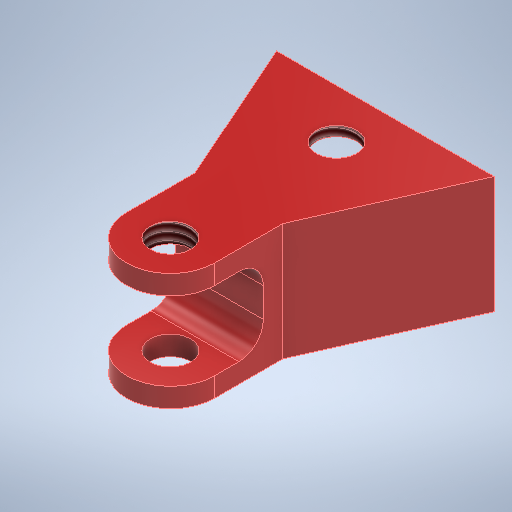
# Autodesk Inventor part: Fixation_rotule_axe_centrale
Saved by Autodesk Inventor 2026.2 (Build 302298010, 298A)
## iProperties
Created: 2026-03-16
Part Number: Fixation_rotule_axe_centrale
Material: Générique
Document SubType Name: Modeling
Designer: genon
Density: 1 g/cm^3
Appearance: Rouge
Author: genon
Autodesk Inventor part; units mm, degrees
ref_plane "YZ Plane" through (0, 0, 0) normal (1, 0, 0) x (0, 1, 0)
ref_plane "XZ Plane" through (0, 0, 0) normal (0, 1, 0) x (-1, 0, 0)
ref_plane "XY Plane" through (0, 0, 0) normal (0, 0, 1) x (1, 0, 0)
sketch "Esquisse1" plane through (0, 0, 0) normal (0, 1, 0) x (-1, 0, 0)
  line L0 (0, 0) -> (0, -15)
  line L1 (0, -15) -> (9.143, -15)
  line L2 (0, -15) -> (9.143, -15) construction
  line L3 (0, -15) -> (-9.143, -15)
  line L4 (0, 0) -> (2.5, 0)
  line L5 (0, 0) -> (-2.5, 0)
  line L6 (-2.5, 0) -> (-9.143, -15)
  line L7 (2.5, 0) -> (9.143, -15)
  line L8 (2.5, 0) -> (4.5, 0)
  line L9 (9.143, -15) -> (11.143, -15)
  line L10 (11.143, -15) -> (4.5, 0)
  line L11 (-9.143, -15) -> (-11.143, -15)
  line L12 (-2.5, 0) -> (-4.5, 0)
  line L13 (-4.5, 0) -> (-11.143, -15)
  line L14 (0, 0) -> (0, 2)
  line L15 (0, 2) -> (4.5, 2)
  line L16 (4.5, 2) -> (4.5, 0)
  line L17 (0, 2) -> (-4.5, 2)
  line L18 (-4.5, 2) -> (-4.5, 0)
  dimension "d0" = 15
  dimension "d1" = 9.143
  dimension "d2" = 0
  dimension "d3" = 9.143
  dimension "d4" = 2.5
  dimension "d5" = 2.5
  dimension "d7" = 2
  dimension "d8" = 2
  dimension "d9" = 2
  dimension "d10" = 2
  dimension "d11" = 2
  constraints: 38 end point, 8 horizontal, 3 perpendicular, 3 point on line, 1 collinear, 1 vertical
  measures "d0" distance of L0.start L0.end
  measures "d1" distance of L0.end L1.end
  measures "d2" distance between parallel lines of L1 L2
  measures "d3" distance of L0.end L3.end
  measures "d4" distance of L0.start L4.end
  measures "d5" distance of L0.start L5.end
  measures "d7" distance of L4.end L8.end
  measures "d8" distance of L2.end L9.end
  measures "d9" distance of L3.end L11.end
  measures "d10" distance of L5.end L12.end
  measures "d11" distance of L0.start L14.end
extrude "Extrusion1" add sketch "Esquisse1" along normal blind 12 contours L14 L15 L16 L8 L4 | L5 L12 L18 L17 L14 | L8 L10 L9 L7 | L6 L11 L13 L12
sketch "Esquisse2" plane through (0, 0, 0) normal (0, -1, 0) x (1, 0, 0)
  line L0 (-2.5, 0) -> (-9.143, -15) projected
  line L1 (-2.5, 0) -> (-9.143, -15)
  line L2 (9.143, -15) -> (2.5, 0) projected
  line L3 (-9.143, -15) -> (9.143, -15)
  line L4 (9.143, -15) -> (2.5, 0)
  line L5 (2.5, 0) -> (-2.5, 0)
  point P0 (0, 0)
  constraints: 8 end point, 2 collinear, 1 horizontal, 1 parallel
extrude "Extrusion2" add sketch "Esquisse2" against normal blind 0.99
sketch "Esquisse3" plane through (0, 12, 0) normal (0, 1, 0) x (1, 0, 0)
  line L0 (2.5, 0) -> (-2.5, 0) projected
  line L1 (2.5, 0) -> (-2.5, 0)
  line L2 (-9.143, 15) -> (-11.143, 15) projected
  line L3 (-2.5, 0) -> (-9.143, 15)
  line L4 (9.143, 15) -> (2.5, 0) projected
  line L5 (-9.143, 15) -> (9.143, 15)
  line L6 (9.143, 15) -> (2.5, 0)
  point P0 (0, 0)
  constraints: 8 end point, 1 collinear, 1 parallel
extrude "Extrusion3" add sketch "Esquisse3" against normal blind 0.99
sketch "Esquisse4" plane through (0, 12, 0) normal (0, 1, 0) x (1, 0, 0)
  line L0 (0, 0) -> (0, 15)
  line L1 (11.143, 15) -> (-11.143, 15) projected
  line L2 (0, 0) -> (0, 10)
  line L3 (0, 10) -> (0, 20)
  dimension "d18" = 10
  dimension "d19" = 10
  constraints: 6 end point, 2 coincident, 2 point on line, 1 midpoint
  measures "d18" distance of L0.start L2.end
  measures "d19" distance of L2.end L3.end
hole "Perçage1" at (0, 12, -10) at (0, 12, -20) direction (0, -1, 0) diameter 4.134 end through all thread size "M5x0.8" class "6H" standard "ISO Metric profile"
sketch "Esquisse5" plane through (0, 12, 0) normal (0, 1, 0) x (1, 0, 0)
  line L0 (-4.5, -2) -> (4.5, -2) projected
  line L1 (-4.5, -2) -> (-4.5, -7)
  line L2 (-4.5, -7) -> (4.5, -7)
  line L3 (4.5, -7) -> (4.5, -2)
  arc A0 (-4.5, -7) -> (4.5, -7) centre (0, -7) ccw
  point P0 (0, 0)
  dimension "d27" = 5
  constraints: 6 end point, 2 perpendicular, 2 point on circle, 1 centre point, 1 midpoint, 1 vertical
  measures "d27" distance of L0.start L1.end
extrude "Extrusion4" add sketch "Esquisse5" against normal blind 2
fillet "Congé1" radius 2.5 1 edges at (0, 10, 2)
sketch "Esquisse7" plane through (0, 12, 0) normal (0, 1, 0) x (1, 0, 0)
  line L0 (4.5, -4.5) -> (-4.5, -4.5) projected
  line L1 (0, -4.5) -> (0, -7.0145)
  point P0 (0, 0)
  dimension "d43" = 2.5145
  constraints: 2 end point, 1 coincident, 1 midpoint
  measures "d43" distance of L1.start L1.end
sketch "Esquisse8" plane through (0, 0, 0) normal (0, -1, 0) x (1, 0, 0)
  line L0 (-4.5, 2) -> (4.5, 2) projected
  line L1 (-4.5, 7) -> (-4.5, 2)
  line L2 (4.5, 7) -> (4.5, 0) projected
  line L3 (4.5, 2) -> (4.5, 7)
  line L4 (-4.5, 2) -> (4.5, 2)
  arc A0 (4.5, 7) -> (-4.5, 7) centre (0, 0.3856) ccw
  arc A1 (4.5, 7) -> (-4.5, 7) centre (0, 7) ccw projected
  line L5 (-4.5, 0) -> (-4.5, 7) projected
  point P0 (0, 0)
  constraints: 6 end point, 2 collinear, 2 point on circle, 1 centre point
extrude "Extrusion5" add sketch "Esquisse8" against normal blind 2
fillet "Congé2" radius 2.5 1 edges at (0, 2, 2)
hole "Perçage2" at (0, 12, 7.0145) direction (0, -1, 0) diameter 4.134 end through all thread size "M5x0.8" class "6H" standard "ISO Metric profile"
